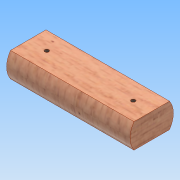
# Autodesk Inventor part: Top_Lever Handle
Saved by Autodesk Inventor 2018.1 (Build 221171000, 171)
## iProperties
Created: 2019-03-23
Part Number: Top_Lever Handle
Material: Wood (Oak)
Document SubType Name: Modeling
Designer: James
Density: 0.76 g/cm^3
Appearance: White Oak - Natural Medium Gloss
Author: James
Autodesk Inventor part; units mm, degrees
ref_plane "YZ Plane" through (0, 0, 0) normal (1, 0, 0) x (0, 1, 0)
ref_plane "XZ Plane" through (0, 0, 0) normal (0, 1, 0) x (-1, 0, 0)
ref_plane "XY Plane" through (0, 0, 0) normal (0, 0, 1) x (1, 0, 0)
sketch "Sketch1" plane through (0, 0, 0) normal (0, 0, 1) x (1, 0, 0)
  line L0 (0, 0) -> (100, 0)
  line L1 (100, 0) -> (100, 17.5)
  line L2 (100, 17.5) -> (0, 17.5)
  line L3 (0, 17.5) -> (0, 0)
  dimension "d0" = 100
  dimension "d1" = 17.5
  constraints: 8 end point, 2 parallel, 1 horizontal, 1 perpendicular
  measures "d0" distance of L1.end L2.end
  measures "d1" distance of L0.end L1.end
revolve "Revolution1" add sketch "Sketch1" angle 360 about axis through (0, 0, 0) along (1, 0, 0)
sketch "Sketch2" plane through (100, 0, 0) normal (1, 0, 0) x (0, 0, -1)
  line L0 (-22.6333, 22.279) -> (-10, 22.279)
  line L1 (-10, 22.279) -> (-10, -22.279)
  line L2 (-10, -22.279) -> (-22.6333, -22.279)
  line L3 (-22.6333, -22.279) -> (-22.6333, 22.279)
  line L4 (10, 22.279) -> (22.1679, 22.279)
  line L5 (22.1679, 22.279) -> (22.1679, -28.0835)
  line L6 (22.1679, -28.0835) -> (10, -28.0835)
  line L7 (10, -28.0835) -> (10, 22.279)
  circle A0 centre (0, 0) radius 17.5 projected
  dimension "d3" = 50.3625
  dimension "d4" = 44.558
  dimension "d5" = 20
  dimension "d6" = 10
  dimension "d7" = 22.279
  dimension "d8" = 12.1679
  dimension "d9" = 12.6333
  dimension "d22" = 35
  constraints: 16 end point, 4 parallel, 2 horizontal, 2 perpendicular, 1 point on line
  measures "d3" distance of L4.end L5.end
  measures "d4" distance of L2.end L0.start
  measures "d5" distance between parallel lines of L7 L1
  measures "d6" distance from line of L7 point (0, 0)
  measures "d7" distance from line of point (0, 0) L0
  measures "d8" distance of L4.start L4.end
  measures "d9" distance of L0.start L0.end
  measures "d22" diameter of A0
extrude "Extrusion1" cut sketch "Sketch2" against normal through all contours L0 L1 A0 L2 L3 | L1 A0 | A0 L7 | L7 L4 L5 L6 A0
sketch "Sketch3" plane through (100, -14.3614, 10) normal (0, 0, 1) x (1, 0, 0)
  line L0 (0, 28.7228) -> (0, 0) projected
  line L1 (-100, 0) -> (-100, 28.7228) projected
  point P0 (-100, 14.3614)
  point P1 (-85, 14.3614)
  point P2 (-15, 14.3614)
  point P3 (0, 14.3614)
  dimension "d12" = 15
  dimension "d13" = 15
  dimension "d14" = 70
  constraints: 2 horizontal alignment, 1 midpoint
  measures "d12" distance from line of point (-15, 14.361) L0
  measures "d13" distance from line of L1 point (-85, 14.361)
  measures "d14" distance of point (-15, 14.361) point (-85, 14.361)
hole "Hole1" at (15, 0, 10) at (85, 0, 10) direction (0, 0, -1) diameter 3.302 end through all thread size "8-32 UNC" class "2B" standard "ANSI Unified Screw Threads"
equation "\"d6\" = 0.5 * d5"
equation "\"d7\" = 0.5 * d4"
equation "\"d13\" = d12"
body "Solid1"
